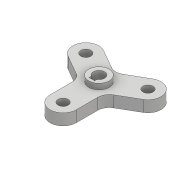
# Autodesk Inventor part: carrier2
Saved by Autodesk Inventor 2018 (Build 220112000, 112)
## iProperties
Created: 2019-12-31
Part Number: carrier2
Material: 一般
Document SubType Name: Modeling
Designer: louis
Density: 1 g/cm^3
Appearance: 預設
Author: louis
Autodesk Inventor part; units mm, degrees
ref_plane "YZ Plane" through (0, 0, 0) normal (1, 0, 0) x (0, 1, 0)
ref_plane "XZ Plane" through (0, 0, 0) normal (0, 1, 0) x (-1, 0, 0)
ref_plane "XY Plane" through (0, 0, 0) normal (0, 0, 1) x (1, 0, 0)
sketch "草圖1" plane through (0, 0, 0) normal (0, 0, 1) x (1, 0, 0)
  line L0 (0, 0) -> (-27.453, 15.85) construction
  line L1 (0, 0) -> (0, -31.7) construction
  circle A0 centre (27.453, 15.85) radius 4.5
  circle A1 centre (0, -31.7) radius 4.5
  circle A2 centre (-27.453, 15.85) radius 4.5
  line L2 (-21.703, 25.8093) -> (-5.0753, 16.2093)
  arc A3 (-5.0753, 16.2093) -> (5.0753, 16.2093) centre (0, 25) ccw
  line L3 (5.0753, 16.2093) -> (21.703, 25.8093)
  line L4 (21.703, 25.8093) -> (21.703, 25.8093)
  arc A4 (33.203, 5.8907) -> (21.703, 25.8093) centre (27.453, 15.85) ccw
  line L5 (33.203, 5.8907) -> (16.5753, -3.7093)
  arc A5 (16.5753, -3.7093) -> (11.5, -12.5) centre (21.6506, -12.5) ccw
  line L6 (11.5, -12.5) -> (11.5, -31.7)
  arc A6 (-11.5, -31.7) -> (11.5, -31.7) centre (0, -31.7) ccw
  line L7 (-11.5, -31.7) -> (-11.5, -12.5)
  arc A7 (-11.5, -12.5) -> (-16.5753, -3.7093) centre (-21.6506, -12.5) ccw
  line L8 (-16.5753, -3.7093) -> (-33.203, 5.8907)
  arc A8 (-21.703, 25.8093) -> (-33.203, 5.8907) centre (-27.453, 15.85) ccw
  line L9 (0, 0) -> (27.453, 15.85) construction
  circle A9 centre (0, 0) radius 8
  dimension "d0" = 31.7
  dimension "d4" = 120
  dimension "d5" = 31.7
  dimension "d6" = 9
  dimension "d7" = 9
  dimension "d8" = 9
  dimension "d9" = 7
  dimension "d10" = 7
  dimension "d11" = 7
  dimension "d12" = 31.7
  dimension "d13" = 120
  dimension "d35" = 25
  dimension "d38" = 16
  constraints: 20 end point, 12 point on circle, 12 tangent, 10 centre point, 4 equal length, 4 parallel, 3 coincident, 3 concentric, 1 vertical
  measures "d0" distance of L0.start L0.end
  measures "d5" distance of L0.start L1.end
  measures "d6" diameter of A2
  measures "d7" diameter of A0
  measures "d8" diameter of A1
  measures "d9" radial gap between concentric circles of A8 A2
  measures "d10" radial gap between concentric circles of A4 A0
  measures "d11" radial gap between concentric circles of A6 A1
  measures "d12" distance of L0.start L9.end
  measures "d35" distance of L0.start A3.centre
  measures "d38" diameter of A9
extrude "擠出1" add sketch "草圖1" along normal blind 10 contours L2 A3 L3 A4 L5 A5 L6 A6 L7 A7 L8 A8 | A9
sketch "草圖2" plane through (0, 0, 10) normal (0, 0, 1) x (1, 0, 0)
  circle A0 centre (0, 0) radius 5
  circle A1 centre (0, 0) radius 9
  line L0 (-2.5, -6.3301) -> (2.5, -6.3301)
  line L1 (-2.5, -6.3301) -> (-2.5, -4.3301)
  line L2 (2.5, -6.3301) -> (2.5, -4.3301)
  dimension "d41" = 10
  dimension "d42" = 18
  dimension "d45" = 5
  dimension "d46" = 2
  constraints: 6 end point, 2 centre point, 2 coincident, 2 parallel, 2 point on circle, 1 horizontal, 1 vertical
  measures "d41" diameter of A0
  measures "d42" diameter of A1
  measures "d45" distance of L0.start L0.end
  measures "d46" distance of L0.start L1.end
extrude "擠出2" cut sketch "草圖2" against normal through all contours A0 | A0 L2 L0 L1
extrude "擠出3" add sketch "草圖2" along normal blind 5
equation "\"d0\" = d5"
equation "\"d6\" = d8"
equation "\"d7\" = d8"
equation "\"d10\" = d9"
equation "\"d11\" = d9"
equation "\"d12\" = d5"
